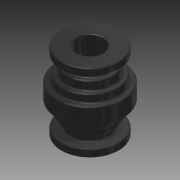
# Autodesk Inventor part: lastik
Saved by Autodesk Inventor 2015 SP1 (Build 190203100, 203)
## iProperties
Created: 2014-11-06
Part Number: lastik
Material: Rubber, Silicone
Document SubType Name: Modeling
Designer: mozata
Density: 1.25 g/cm^3
Appearance: Rubber - Black - Version 1.1
Mass: 3.11318 g
Surface Area: 22.8816 cm^2
Volume: 2.49054 cm^3
Author: mozata
Autodesk Inventor part; units mm, degrees
ref_plane "YZ Plane" through (0, 0, 0) normal (1, 0, 0) x (0, 1, 0)
ref_plane "XZ Plane" through (0, 0, 0) normal (0, 1, 0) x (-1, 0, 0)
ref_plane "XY Plane" through (0, 0, 0) normal (0, 0, 1) x (1, 0, 0)
sketch "Sketch1" plane through (0, 0, 0) normal (0, 0, 1) x (1, 0, 0)
  circle A0 centre (0, 0) radius 9
  circle A1 centre (0, 0) radius 5
  dimension "d0" = 18
  dimension "d3" = 10
  constraints: 2 centre point, 2 coincident
  measures "d0" diameter of A0
  measures "d3" diameter of A1
extrude "Extrusion1" add sketch "Sketch1" along normal blind 2.25
sketch "Sketch2" plane through (0, 0, 2.25) normal (0, 0, 1) x (1, 0, 0)
  circle A0 centre (0, 0) radius 7.5
  circle A1 centre (0, 0) radius 3.5
  dimension "d4" = 15
  dimension "d5" = 7
  constraints: 2 centre point, 2 coincident
  measures "d4" diameter of A0
  measures "d5" diameter of A1
extrude "Extrusion2" add sketch "Sketch2" along normal blind 2
sketch "Sketch3" plane through (0, 0, 4.25) normal (0, 0, 1) x (1, 0, 0)
  circle A0 centre (0, 0) radius 3.5 projected
  circle A1 centre (0, 0) radius 6.25
  dimension "d8" = 12.5
  constraints: 1 centre point, 1 coincident
  measures "d8" diameter of A1
extrude "Extrusion3" add sketch "Sketch3" along normal blind 2.25
sketch "Sketch4" plane through (0, 0, 6.5) normal (0, 0, 1) x (1, 0, 0)
  circle A0 centre (0, 0) radius 3.5 projected
  circle A1 centre (0, 0) radius 5
  dimension "d11" = 10
  constraints: 1 centre point, 1 coincident
  measures "d11" diameter of A1
extrude "Extrusion4" add sketch "Sketch4" along normal blind 2
sketch "Sketch5" plane through (0, 0, 8.5) normal (0, 0, 1) x (1, 0, 0)
  circle A0 centre (0, 0) radius 7.8
  circle A1 centre (0, 0) radius 3.5 projected
  dimension "d14" = 15.6
  constraints: 1 centre point, 1 coincident
  measures "d14" diameter of A0
extrude "Extrusion5" add sketch "Sketch5" along normal blind 2
fillet "Fillet1" radius 0.3 12 edges at (-7.5, 0, 2.25) (-7.5, 0, 4.25) (-6.25, 0, 4.25) (-6.25, 0, 6.5) (-5, 0, 6.5) (-5, 0, 8.5) (-7.8, 0, 8.5) (-7.8, 0, 10.5) (-9, 0, 2.25) (-3.5, 0, 2.25) (-5, 0, 2.25) (-3.5, 0, 10.5)
mirror "Mirror2" about plane through (0, 0, 0) normal (0, 0, 1)
body "Solid1"
